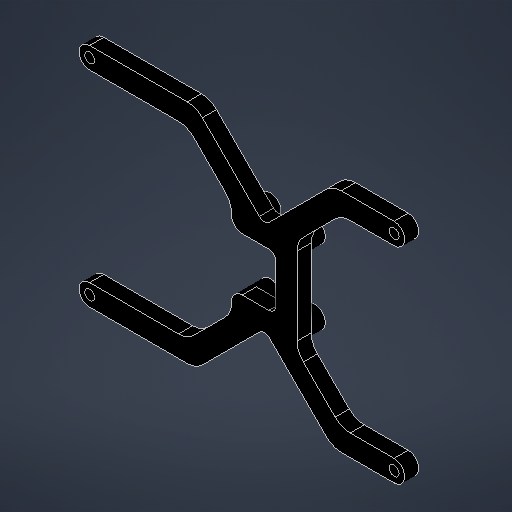
# Autodesk Inventor part: Camera Bracket
Saved by Autodesk Inventor 2026.1 (Build 301233020, 233B)
## iProperties
Created: 2026-04-07
Part Number: Camera Bracket
Material: Generic
Document SubType Name: Modeling
Designer: Bahaa
Mass: 5.96086 g
Surface Area: 52.9976 cm^2
Volume: 5.96086 cm^3
Density: 1 g/cm^3
Appearance: Default(1)
Author: Bahaa
Autodesk Inventor part; units mm, degrees
ref_plane "YZ Plane" through (0, 0, 0) normal (1, 0, 0) x (0, 1, 0)
ref_plane "XZ Plane" through (0, 0, 0) normal (0, 1, 0) x (-1, 0, 0)
ref_plane "XY Plane" through (0, 0, 0) normal (0, 0, 1) x (1, 0, 0)
sketch "Sketch1" plane through (0, 0, 0) normal (0, 1, 0) x (-1, 0, 0)
  line L0 (12, 12.5) -> (-12, 12.5) construction
  line L1 (-12, 12.5) -> (-12, -12.5) construction
  line L2 (-12, -12.5) -> (12, -12.5) construction
  line L3 (12, -12.5) -> (12, 12.5) construction
  line L4 (12, 12.5) -> (-12, -12.5) construction
  line L5 (-12, 12.5) -> (12, -12.5) construction
  line L6 (12, 0) -> (-12, 0) construction
  line L7 (0, 12.5) -> (0, -12.5) construction
  circle A0 centre (2.5, 10.5) radius 3
  circle A1 centre (2.5, -10.5) radius 3
  circle A2 centre (-10, 10.5) radius 3
  circle A3 centre (-10, -10.5) radius 3
  line L8 (2.5, 10.5) -> (-10.08, 10.5) construction
  line L9 (2.5, 13.5) -> (-10.08, 13.5)
  line L10 (-10.08, 7.5) -> (2.5, 7.5)
  arc A4 (2.5, 7.5) -> (2.5, 13.5) centre (2.5, 10.5) ccw
  line L11 (2.5, -13.5) -> (-10.08, -13.5)
  line L12 (-10.08, -7.5) -> (2.5, -7.5)
  line L13 (-7, 10.5) -> (-7, -10.5)
  line L14 (0, 29) -> (45.6, 29) construction
  line L15 (45.6, 29) -> (45.6, -29) construction
  line L16 (45.6, -29) -> (0, -29) construction
  line L17 (0, -29) -> (0, 29) construction
  line L18 (0, 29) -> (45.6, -29) construction
  line L19 (45.6, 29) -> (0, -29) construction
  line L20 (0, 29) -> (-40.4, 29) construction
  line L21 (-40.4, 29) -> (-40.4, -29) construction
  line L22 (-40.4, -29) -> (0, -29) construction
  line L23 (0, -29) -> (0, 29) construction
  line L24 (0, 29) -> (-40.4, -29) construction
  line L25 (-40.4, 29) -> (0, -29) construction
  circle A5 centre (45.6, 29) radius 1.4
  circle A6 centre (45.6, -29) radius 1.4
  line L26 (0, 0) -> (0, -7.5) construction
  circle A7 centre (-40.4, 29) radius 1.4
  circle A8 centre (-40.4, -29) radius 1.4
  circle A9 centre (45.6, 29) radius 3
  line L27 (-0.5, 32) -> (5.5, 32)
  line L28 (5.5, 32) -> (5.5, 26) construction
  line L29 (5.5, 26) -> (-0.5, 26) construction
  line L30 (-0.5, 26) -> (-0.5, 32)
  line L31 (-0.5, 32) -> (5.5, 26) construction
  line L32 (5.5, 32) -> (-0.5, 26) construction
  line L33 (2.5, 10.5) -> (2.5, -10.5) construction
  line L34 (45.6, 32) -> (5.5, 32)
  line L35 (45.6, 26) -> (18, 26)
  line L36 (5.5, 13.5) -> (5.5, 10.5)
  line L37 (-0.5, 26) -> (-0.5, 10.5)
  line L38 (-13, 32) -> (-7, 32)
  line L39 (-7, 32) -> (-7, 26)
  line L40 (-7, 26) -> (-13, 26) construction
  line L41 (-13, 26) -> (-13, 32) construction
  line L42 (-13, 32) -> (-7, 26) construction
  line L43 (-7, 32) -> (-13, 26) construction
  line L44 (-13, 10.5) -> (-13, -10.5)
  line L45 (-7, 26) -> (-7, 10.5)
  line L46 (-13, 13.5) -> (-13, 10.5)
  circle A10 centre (-40.4, 29) radius 3
  line L47 (-13, 32) -> (-40.4, 32)
  line L48 (-25.5, 26) -> (-40.4, 26)
  line L49 (0, -29) -> (45.6, -29) construction
  line L50 (45.6, -29) -> (45.6, 29) construction
  line L51 (0, 29) -> (0, -29) construction
  line L52 (0, -29) -> (45.6, 29) construction
  line L53 (45.6, -29) -> (0, 29) construction
  line L54 (0, -29) -> (-40.4, -29) construction
  line L55 (-40.4, -29) -> (-40.4, 29) construction
  line L56 (0, 29) -> (0, -29) construction
  line L57 (0, -29) -> (-40.4, 29) construction
  line L58 (-40.4, -29) -> (0, 29) construction
  circle A11 centre (45.6, -29) radius 1.4
  circle A12 centre (-40.4, -29) radius 1.4
  circle A13 centre (45.6, -29) radius 3
  line L59 (-0.5, -32) -> (5.5, -32)
  line L60 (5.5, -32) -> (5.5, -26) construction
  line L61 (5.5, -26) -> (-0.5, -26) construction
  line L62 (-0.5, -26) -> (-0.5, -32)
  line L63 (-0.5, -32) -> (5.5, -26) construction
  line L64 (5.5, -32) -> (-0.5, -26) construction
  line L65 (45.6, -32) -> (5.5, -32)
  line L66 (45.6, -26) -> (18, -26)
  line L67 (5.5, -13.5) -> (5.5, -10.5)
  line L68 (-0.5, -26) -> (-0.5, -10.5)
  line L69 (-13, -32) -> (-7, -32)
  line L70 (-7, -32) -> (-7, -26)
  line L71 (-7, -26) -> (-13, -26) construction
  line L72 (-13, -26) -> (-13, -32) construction
  line L73 (-13, -32) -> (-7, -26) construction
  line L74 (-7, -32) -> (-13, -26) construction
  line L75 (-7, -26) -> (-7, -10.5)
  line L76 (-13, -13.5) -> (-13, -10.5)
  circle A14 centre (-40.4, -29) radius 3
  line L77 (-13, -32) -> (-40.4, -32)
  line L78 (-25.5, -26) -> (-40.4, -26)
  line L79 (18, 26) -> (5.5, 13.5)
  line L80 (5.5, -13.5) -> (18, -26)
  line L81 (-13, -13.5) -> (-25.5, -26)
  line L82 (-13, 13.5) -> (-25.5, 26)
  line L83 (15.5147, 32) -> (-2.9853, 13.5)
  line L84 (15.5147, -32) -> (-2.9853, -13.5)
  line L85 (-4.5147, 13.5) -> (-23.0147, 32)
  line L86 (-4.5147, -13.5) -> (-23.0147, -32)
  point P0 (0, 0)
  point P1 (22.8, 0)
  point P2 (0, 0)
  point P3 (-20.2, 0)
  point P4 (2.5, 29)
  point P5 (-10, 29)
  point P6 (2.5, -29)
  point P7 (-10, -29)
  point P8 (-7, -13.5)
  point P9 (-0.5, -13.5)
  point P10 (5.5, -10.5)
  point P11 (2.5, -7.5)
  point P12 (-7, -7.5)
  point P13 (-7, 7.5)
  point P14 (2.5, 7.5)
  point P15 (5.5, 10.5)
  point P16 (-0.5, 13.5)
  point P17 (-7, 13.5)
  point P18 (-0.5, 15.9853)
  point P19 (11.75, 19.75)
  point P20 (-0.5, -15.9853)
  point P21 (-7, 15.9853)
  point P22 (-7, -15.9853)
  point P23 (-0.5, -15.9853)
  dimension "d7" = 6
  dimension "d0" = 24
  dimension "d1" = 25
  dimension "d3" = 2
  dimension "d4" = 2
  dimension "d5" = 9.5
  dimension "d6" = 2
  dimension "d8" = 6
  dimension "d9" = 6
  dimension "d10" = 45.6
  dimension "d11" = 58
  dimension "d12" = 40.4
  dimension "d13" = 58
  dimension "d14" = 2.8
  dimension "d15" = 2.8
  dimension "d16" = 6
  dimension "d17" = 6
  dimension "d18" = 6
  dimension "d19" = 6
  dimension "d20" = 6
  dimension "d21" = 6
  dimension "d24" = 12.5
  dimension "d25" = 12.5
  dimension "d26" = 12.5
  dimension "d27" = 12.5
  dimension "d28" = 12.5
  dimension "d29" = 12.5
  dimension "d30" = 12.5
  dimension "d31" = 12.5
  dimension "d33" = 6
  dimension "d34" = 6
  dimension "d35" = 6
  constraints: 176 end point, 40 symmetric about line, 38 point on line, 19 midpoint, 15 parallel, 15 point on circle, 14 centre point, 10 coincident, 8 tangent, 6 horizontal, 5 perpendicular, 1 vertical, 11 other
  measures "d0" distance of L2.end L1.end
  measures "d1" distance of L1.end L0.end
  measures "d3" distance from line of L1 point (-10, 10.5)
  measures "d4" distance from line of L0 point (-10, 10.5)
  measures "d5" distance from line of L3 point (2.5, 10.5)
  measures "d6" distance from line of L0 point (2.5, 10.5)
  measures "d8" diameter of A2
  measures "d9" distance between parallel lines of L10 L9
  measures "d10" distance of L15.end L16.end
  measures "d11" distance of L14.end L15.end
  measures "d12" distance of L22.end L21.end
  measures "d13" distance of L21.end L20.end
  measures "d14" diameter of A5
  measures "d15" diameter of A7
  measures "d16" diameter of A9
  measures "d17" distance of L28.end L29.end
  measures "d18" distance of L27.end L28.end
  measures "d19" distance of L39.end L40.end
  measures "d20" distance of L38.end L39.end
  measures "d21" diameter of A10
  measures "d24" distance of L35.end L28.end
  measures "d25" distance of L36.start L28.end
  measures "d26" distance of L67.start L61.start
  measures "d27" distance of L66.end L61.start
  measures "d28" distance of L76.start L71.end
  measures "d29" distance of L78.start L71.end
  measures "d30" distance of L46.start L40.end
  measures "d31" distance of L48.start L40.end
  measures "d33" distance from line of point (11.75, 19.75) L83
  measures "d34" distance between parallel lines of L82 L85
  measures "d35" distance between parallel lines of L81 L86
extrude "Extrusion1" add sketch "Sketch1" against normal blind 4 contours A0 | A0 L9 L37 L83 L34 A9 L35 L79 L36 | A0 L37 L9 | L10 L13 L45 L9 L37 A0 | L9 L83 L37 | A2 L46 L82 L48 A10 L47 L85 L45 L9 | A2 | L12 L13 A3 | L13 L12 A3 L44 A2 L10 | L10 A2 L13 | A2 L9 L45 | L12 A1 L68 L11 L75 L13 | A9 | L9 L45 L85 | A3 L75 L11 | A3 | A1 | A3 L11 L75 L86 L77 A14 L78 L81 L76 | L67 L80 L66 A13 L65 L84 L68 L11 A1 | A1 L11 L68 | L11 L86 L75 | L68 L84 L11 | A10 | A14 | A13
extrude "Extrusion2" add sketch "Sketch1" along normal blind 4 contours A0 | A2 | A3 | A1
fillet "Fillet1" radius 6 12 edges at (-18, -2, 26) (-18, -2, -26) (25.5, -2, 26) (25.5, -2, -26) (23.0147, -2, 32) (23.0147, -2, -32) (-15.5147, -2, 32) (-15.5147, -2, -32) (-5.5, -2, 13.5) (-5.5, -2, -13.5) (13, -2, 13.5) (13, -2, -13.5)
fillet "Fillet2" radius 2 6 edges at (7, -2, 7.5) (7, -2, -7.5) (4.5147, -2, 13.5) (2.9853, -2, 13.5) (2.9853, -2, -13.5) (4.5147, -2, -13.5)
sketch "Sketch2" plane through (-2.5, 4, 10.5) normal (0, 1, 0) x (1, 0, 0)
  circle A0 centre (12.5, 0) radius 3 projected
  circle A1 centre (0, 21) radius 3 projected
  circle A2 centre (12.5, 21) radius 3 projected
  circle A3 centre (0, 0) radius 3 projected
  point P0 (2.5, 10.5)
hole "Hole1" at (-2.5, 4, 10.5) at (-2.5, 4, -10.5) at (10, 4, -10.5) at (10, 4, 10.5) direction (0, -1, 0) diameter 3.3 depth 4
equation "\"d8\" = d7"
equation "\"d9\" = d7"
equation "\"d15\" = d14"
equation "\"d17\" = d7"
equation "\"d18\" = d7"
equation "\"d19\" = d7"
equation "\"d20\" = d7"
equation "\"d21\" = d7"
equation "\"d25\" = d24"
equation "\"d26\" = d24"
equation "\"d27\" = d26"
equation "\"d28\" = d24"
equation "\"d29\" = d28"
equation "\"d30\" = d24"
equation "\"d31\" = d30"
equation "\"d33\" = d7"
equation "\"d34\" = d7"
equation "\"d35\" = d7"
body "Solid1"
